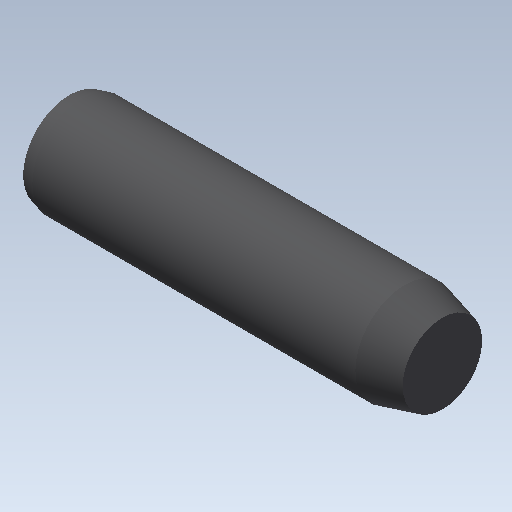
# Autodesk Inventor part: MSVC4-15
Saved by Autodesk Inventor 2020 (Build 240168000, 168)
## iProperties
Created: 2017-05-10
Part Number: MSVC4-15
Catalog Web Link: www.cadenas.de
Description: MSV, MSVC-Dowel Pins - High Precision
Vendor: MISUMI
Document SubType Name: Modeling
Designer: psAdmin
Manufacturer: MISUMI
Mass: 0.18455 g
Surface Area: 2.06166 cm^2
Volume: 0.18455 cm^3
Density: 1 g/cm^3
Material: Generic
Appearance: PSOLRGB-175-175-175
Category: PARTsolutions
Company: MISUMI
PSOL_IDENT_0: {$CADENAS_DATA\23d-libs\misumi\metric\28_keys_magnets\msv.prj},155 {VTYP=3D},{NB=MSVC4-15},{LINA=MSV
PSOL_IDENT_1: C4-15},{NN=MSV, MSVC},{DATE=24.04.2017 10:16:56},{GEOMDATE=31.01.2012},{VERSION=},{LINEID=20},{LINES
PSOL_IDENT_2: UBID=-1},{WBVAR=D,L}  {NB=MSVC4-15},{LINA=MSVC4-15},{KT=DUMMY},{PN=MSVC4-15},{TYPE=MSVC},{MAT=440C S
PSOL_IDENT_3: tainless Steel},{HARD=58HRC~},{D=4.0},{DALG=[1,1.5,2,3,4,5,6,8,10]},{L=15},{LALG=[8,10,15,20,25,30]}
PSOL_IDENT_4: ,{LL1=1.5},{LL2=0.5}
NN: MSV, MSVC
NT: Dowel Pins - High Precision
NB: MSVC4-15
NBSYN: $PN.
LINA: MSVC4-15
PN: MSVC4-15
MAT: 440C Stainless Steel
HARD: 58HRC~
D: 4.0
L: 15
LL1: 1.5
LL2: 0.5
SUPPLIER: MISUMI
ARTICLENO: MSVC4-15
BOMINFO: MSVC4-15
CREATOR: CADENAS GmbH
Title: MSVC4-15
Author: Cadenas PARTsolutions
Comments: Dowel Pins - High Precision
Autodesk Inventor part; units mm, degrees
ref_plane "YZ Plane" through (0, 0, 0) normal (1, 0, 0) x (0, 1, 0)
ref_plane "XZ Plane" through (0, 0, 0) normal (0, 1, 0) x (-1, 0, 0)
ref_plane "XY Plane" through (0, 0, 0) normal (0, 0, 1) x (1, 0, 0)
sketch "Sketch_1" plane through (0, 0, 0) normal (0, 0, 1) x (1, 0, 0)
  line L0 (7.5, 0) -> (-7.5, 0)
  line L1 (-7.5, 0) -> (-7.5, 1.866)
  line L2 (-7.5, 1.866) -> (-7, 2)
  line L3 (-7, 2) -> (6, 2)
  line L4 (6, 2) -> (7.5, 1.5981)
  line L5 (7.5, 1.5981) -> (7.5, 0)
  line L6 (7.5, 0) -> (-7.5, 0)
  constraints: 14 end point
revolve "Revolution1" add sketch "Sketch_1" angle 360 about axis through (7.5, 0, 0) along (1, 0, 0)
body "Solid1"
